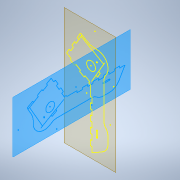
# Autodesk Inventor part: wooden_internal
Saved by Autodesk Inventor 2020 (Build 240168000, 168)
## iProperties
Created: 2019-07-29
Part Number: wooden_internal
Material: Generic
Document SubType Name: Modeling
Designer: erwin
Density: 1 g/cm^3
Appearance: Default
Author: erwin
Autodesk Inventor part; units mm, degrees
ref_plane "YZ Plane" through (0, 0, 0) normal (1, 0, 0) x (0, 1, 0)
ref_plane "XZ Plane" through (0, 0, 0) normal (0, 1, 0) x (-1, 0, 0)
ref_plane "XY Plane" through (0, 0, 0) normal (0, 0, 1) x (1, 0, 0)
ref_plane "Work Plane1" through (0, 0, 0) normal (0, 0, 1) x (1, 0, 0)
sketch "Sketch1" plane through (0, 0, 0) normal (0, 0, 1) x (1, 0, 0)
  circle A0 centre (68.2595, 214.6541) radius 4 projected
  line L0 (64.2595, -185.3459) -> (64.2595, -225.3459) projected
  arc A1 (72.2595, -185.3459) -> (64.2595, -185.3459) centre (68.2595, -185.3459) ccw projected
  line L1 (72.2595, -225.3459) -> (72.2595, -185.3459) projected
  arc A2 (64.2595, -225.3459) -> (72.2595, -225.3459) centre (68.2595, -225.3459) ccw projected
  line L2 (-101.2595, 230.5421) -> (-90.8671, 224.5421) projected
  line L3 (-90.8671, 224.5421) -> (-108.8671, 193.3652) projected
  line L4 (-108.8671, 193.3652) -> (-119.2595, 199.3652) projected
  line L5 (-137.2595, 168.1883) -> (-119.2595, 199.3652) projected
  line L6 (-137.2595, 168.1883) -> (-106.0825, 150.1883) projected
  line L7 (-106.0825, 150.1883) -> (-112.0825, 139.796) projected
  line L8 (-80.9056, 121.796) -> (-112.0825, 139.796) projected
  line L9 (-80.9056, 121.796) -> (-74.9056, 132.1883) projected
  line L10 (-74.9056, 132.1883) -> (-43.7287, 114.1883) projected
  line L11 (-43.7287, 114.1883) -> (-49.7287, 103.796) projected
  line L12 (-18.5518, 85.796) -> (-49.7287, 103.796) projected
  line L13 (-18.5518, 85.796) -> (-12.5518, 96.1883) projected
  line L14 (-12.5518, 96.1883) -> (18.6251, 78.1883) projected
  line L15 (18.6251, 78.1883) -> (12.6251, 67.796) projected
  line L16 (23.2595, 61.6562) -> (12.6251, 67.796) projected
  line L17 (23.2595, -7.001) -> (23.2595, 61.6562) projected
  line L18 (23.2595, -7.001) -> (35.2595, -7.001) projected
  line L19 (35.2595, -7.001) -> (35.2595, -43.001) projected
  line L20 (35.2595, -43.001) -> (23.2595, -43.001) projected
  line L21 (23.2595, -79.001) -> (23.2595, -43.001) projected
  line L22 (23.2595, -79.001) -> (35.2595, -79.001) projected
  line L23 (35.2595, -79.001) -> (35.2595, -115.001) projected
  line L24 (35.2595, -115.001) -> (23.2595, -115.001) projected
  line L25 (23.2595, -151.001) -> (23.2595, -115.001) projected
  line L26 (23.2595, -151.001) -> (35.2595, -151.001) projected
  line L27 (35.2595, -151.001) -> (35.2595, -187.001) projected
  line L28 (35.2595, -187.001) -> (23.2595, -187.001) projected
  line L29 (23.2595, -223.001) -> (23.2595, -187.001) projected
  line L30 (23.2595, -223.001) -> (35.2595, -223.001) projected
  line L31 (35.2595, -223.001) -> (35.2595, -259.001) projected
  line L32 (35.2595, -259.001) -> (23.2595, -259.001) projected
  line L33 (23.2595, -295.001) -> (23.2595, -259.001) projected
  line L34 (23.2595, -295.001) -> (35.2595, -295.001) projected
  line L35 (35.2595, -295.001) -> (35.2595, -331.001) projected
  line L36 (105.7595, -290.2979) -> (35.2595, -331.001) projected
  arc A3 (105.7595, -290.2979) -> (143.2595, -225.3459) centre (68.2595, -225.3459) ccw projected
  line L37 (143.2595, -185.3459) -> (143.2595, -225.3459) projected
  arc A4 (143.2595, -185.3459) -> (125.3012, -136.6505) centre (68.2595, -185.3459) ccw projected
  arc A5 (114.6586, -107.7924) -> (125.3012, -136.6505) centre (159.1055, -107.7924) ccw projected
  line L38 (114.6586, 129.2663) -> (114.6586, -107.7924) projected
  arc A6 (128.1281, 169.4795) -> (114.6586, 129.2663) centre (181.4216, 129.2663) ccw projected
  arc A7 (128.1281, 169.4795) -> (62.9654, 289.467) centre (68.2595, 214.6541) ccw projected
  arc A8 (5.9066, 302.615) -> (62.9654, 289.467) centre (55.9066, 389.2175) ccw projected
  line L39 (-43.2595, 331.001) -> (5.9066, 302.615) projected
  line L40 (-65.2595, 292.8959) -> (-43.2595, 331.001) projected
  line L41 (-65.2595, 292.8959) -> (-54.8671, 286.8959) projected
  line L42 (-54.8671, 286.8959) -> (-72.8671, 255.719) projected
  line L43 (-72.8671, 255.719) -> (-83.2595, 261.719) projected
  line L44 (-101.2595, 230.5421) -> (-83.2595, 261.719) projected
  circle A9 centre (28.2595, 174.6541) radius 30 projected
  line L45 (71.9456, 130.5421) -> (61.5533, 136.5421) projected
  line L46 (61.5533, 136.5421) -> (79.5533, 167.719) projected
  line L47 (79.5533, 167.719) -> (89.9456, 161.719) projected
  line L48 (89.9456, 161.719) -> (71.9456, 130.5421) projected
  line L49 (-32.8671, 325.001) -> (-54.8671, 286.8959) projected
  line L50 (61.5533, 136.5421) -> (30.0629, 81.9992) projected
  line L51 (-12.5518, 96.1883) -> (18.6251, 78.1883) projected
  line L52 (-38.0011, 314.1087) -> (112.6873, 227.1087) projected
  line L53 (-54.8671, 286.8959) -> (-72.8671, 255.719) projected
  line L54 (-74.9056, 132.1883) -> (-43.7287, 114.1883) projected
  line L55 (-38.0011, 314.1087) -> (112.6873, 227.1087) projected
  line L56 (119.5533, 237.001) -> (79.5533, 167.719) projected
  line L57 (-38.8671, 314.6087) -> (-126.8671, 162.1883)
  line L58 (-126.8671, 162.1883) -> (25.5533, 74.1883)
  line L59 (25.5533, 74.1883) -> (113.5533, 226.6087)
  line L60 (113.5533, 226.6087) -> (-38.8671, 314.6087)
  circle A10 centre (-126.8671, 162.1883) radius 15
  circle A11 centre (25.5533, 74.1883) radius 15
  circle A12 centre (28.2595, 174.6541) radius 30
  point P0 (0, 0)
  point P1 (37.3431, 270.6087)
  point P2 (37.3431, 270.6087)
  point P3 (70.5533, 152.1306)
  point P4 (-59.3172, 123.1883)
  point P5 (12.5629, 81.6883)
  point P6 (33.0533, 87.1787)
  point P7 (-119.3671, 175.1787)
  point P8 (-113.8768, 154.6883)
  dimension "d0" = 30
  dimension "d1" = 30
  dimension "d2" = 60
  constraints: 8 end point, 5 midpoint, 3 centre point, 3 coincident, 2 perpendicular, 2 point on line, 1 collinear, 1 parallel
  measures "d0" diameter of A10
  measures "d1" diameter of A11
  measures "d2" diameter of A12
extrude "Extrusion1" add sketch "Sketch1" along normal blind 12 contours A0 | L57 L42 L49 L60 L52 L56 L46 L50 A11 L14 L58 L10 L6 A10 L3
move faces "Move1" translate (-0.5, -0.866, 0) faces at (113.2646, 226.7754, 4) (62.4578, 256.1087, 4) (-38.2898, 314.2754, 4)
equation "\"d1\" = d0"
body "Solid1"
